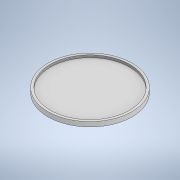
# Autodesk Inventor part: Drainage Base
Saved by Autodesk Inventor 2022 (Build 260153000, 153)
## iProperties
Created: 2021-11-11
Part Number: Drainage Base
Material: Generic
Document SubType Name: Modeling
Designer: aed0019
Density: 1 g/cm^3
Appearance: Default
Author: aed0019
Autodesk Inventor part; units mm, degrees
ref_plane "YZ Plane" through (0, 0, 0) normal (1, 0, 0) x (0, 1, 0)
ref_plane "XZ Plane" through (0, 0, 0) normal (0, 1, 0) x (-1, 0, 0)
ref_plane "XY Plane" through (0, 0, 0) normal (0, 0, 1) x (1, 0, 0)
sketch "Sketch1" plane through (0, 0, 0) normal (0, 1, 0) x (-1, 0, 0)
  circle A0 centre (0, 0) radius 114.3
  circle A1 centre (0, 0) radius 107.95
  line L0 (-63.5, -63.5) -> (63.5, -63.5)
  line L1 (63.5, -63.5) -> (63.5, 63.5)
  line L2 (63.5, 63.5) -> (-63.5, 63.5)
  line L3 (-63.5, 63.5) -> (-63.5, -63.5)
  line L4 (-63.5, -63.5) -> (63.5, 63.5) construction
  line L5 (63.5, -63.5) -> (-63.5, 63.5) construction
  line L6 (57.15, 57.15) -> (57.15, -57.15)
  line L7 (57.15, -57.15) -> (-57.15, -57.15)
  line L8 (-57.15, -57.15) -> (-57.15, 57.15)
  line L9 (-57.15, 57.15) -> (57.15, 57.15)
  dimension "d0" = 228.6
  dimension "d1" = 6.35
  dimension "d2" = 127
  dimension "d3" = 127
  dimension "d4" = 6.35
  constraints: 20 end point, 4 parallel, 2 centre point, 2 midpoint, 2 perpendicular, 1 coincident, 1 horizontal, 3 other
  measures "d0" diameter of A0
  measures "d1" radial gap between concentric circles of A0 A1
  measures "d2" distance of L2.end L1.end
  measures "d3" distance of L1.end L0.end
  measures "d4" distance between parallel lines of L1 L6
extrude "Extrusion1" add sketch "Sketch1" along normal blind 6.35 contours A1
extrude "Extrusion2" add sketch "Sketch1" along normal blind 12.7 contours A0
extrude "Extrusion3" add sketch "Sketch1" along normal blind 6.35 contours L3 L2 L1 L0 | L6 L7 L8 L9
body "Solid1"
